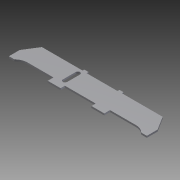
# Autodesk Inventor part: Deslizador
Saved by Autodesk Inventor 2011 (Build 150239000, 239)
## iProperties
Created: 2014-08-04
Part Number: Deslizador
Material: Por defecto
Document SubType Name: Chapa
Designer: amatiasq
Density: 1 g/cm^3
Sheet Metal Rule: Por defecto_mm
Author: amatiasq
Autodesk Inventor part; units mm, degrees
ref_plane "YZ Plane" through (0, 0, 0) normal (1, 0, 0) x (0, 1, 0)
ref_plane "XZ Plane" through (0, 0, 0) normal (0, 1, 0) x (-1, 0, 0)
ref_plane "XY Plane" through (0, 0, 0) normal (0, 0, 1) x (1, 0, 0)
sketch "Boceto1" plane through (0, 0, 0) normal (0, 0, 1) x (1, 0, 0)
  line L0 (0, 5) -> (18, 5)
  line L1 (18, 5) -> (18, 0)
  line L2 (18, 0) -> (33, 0)
  line L3 (33, 0) -> (33, 6.7)
  line L4 (33, 6.7) -> (64, 6.7)
  line L5 (0, 30.4) -> (18, 30.4)
  line L6 (18, 30.4) -> (18, 32.7)
  line L7 (18, 32.7) -> (23, 32.7)
  line L8 (23, 32.7) -> (23, 30.7)
  line L9 (23, 30.7) -> (70.5, 30.7)
  line L10 (80.5, 14.7) -> (70.5, 30.7)
  line L11 (80.5, 14.7) -> (80.5, 2.2)
  line L12 (80.5, 2.2) -> (74, 2.2)
  arc A0 (74, 2.2) -> (64, 6.7) centre (63.2705, -8.2822) ccw
  line L13 (0, 5) -> (-18, 5)
  line L14 (-18, 5) -> (-18, 0)
  line L15 (-18, 0) -> (-33, 0)
  line L16 (-33, 0) -> (-33, 6.7)
  line L17 (-33, 6.7) -> (-64, 6.7)
  line L18 (0, 30.4) -> (-18, 30.4)
  line L19 (-18, 30.4) -> (-18, 32.7)
  line L20 (-18, 32.7) -> (-23, 32.7)
  line L21 (-23, 32.7) -> (-23, 30.7)
  line L22 (-23, 30.7) -> (-70.5, 30.7)
  line L23 (-80.5, 14.7) -> (-70.5, 30.7)
  line L24 (-80.5, 14.7) -> (-80.5, 2.2)
  line L25 (-80.5, 2.2) -> (-74, 2.2)
  arc A1 (-64, 6.7) -> (-74, 2.2) centre (-63.2705, -8.2822) ccw
  line L26 (-25.5, 10.2) -> (-25.5, 25.2)
  line L27 (-20.5, 25.2) -> (-20.5, 10.2)
  arc A2 (-20.5, 25.2) -> (-25.5, 25.2) centre (-23, 25.2) ccw
  arc A3 (-25.5, 10.2) -> (-20.5, 10.2) centre (-23, 10.2) ccw
  point P0 (0, 0)
  dimension "d0" = 18
  dimension "d1" = 15
  dimension "d2" = 6.7
  dimension "d3" = 31
  dimension "d4" = 18
  dimension "d5" = 2.3
  dimension "d6" = 5
  dimension "d7" = 2
  dimension "d8" = 47.5
  dimension "d9" = 12.5
  dimension "d10" = 6.5
  dimension "d11" = 15
  dimension "d12" = 5
  dimension "d13" = 15
  constraints: 56 end point, 8 parallel, 8 point on circle, 4 centre point, 4 perpendicular, 4 tangent, 1 horizontal
  measures "d0" distance of L0.start L0.end
  measures "d1" distance of L1.end L2.end
  measures "d2" distance of L2.end L3.end
  measures "d3" distance of L3.end L4.end
  measures "d4" distance of L5.start L5.end
  measures "d5" distance of L5.end L6.end
  measures "d6" distance of L6.end L7.end
  measures "d7" distance of L7.end L8.end
  measures "d8" distance of L8.end L9.end
  measures "d9" distance of L10.start L11.end
  measures "d10" distance of L11.end L12.end
  measures "d11" radius of A0
  measures "d12" distance of L26.end L27.start
  measures "d13" distance of L26.start L26.end
extrude "Extrusión1" add sketch "Boceto1" along normal blind 2
equation "\"Radio_pliegue\" = Grosor"
equation "\"Anchura_desahogo_plegado\" = Grosor"
equation "\"Profundidad_desahogo_plegado\" = 0.5 * Grosor"
equation "\"Tamaño_destalonado\" = 4 * Grosor"
equation "\"Remanente_mínimo\" = 2 * Grosor"
equation "\"Radiodetransición\" = Radio_pliegue"
equation "\"Tamaño_de_radio_de_Jacobi\" = Radio_pliegue"
equation "\"TamañoSeparación\" = Grosor"
equation "\"Grosor\" = 0.5"
